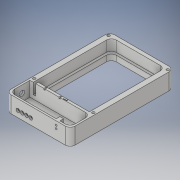
# Autodesk Inventor part: Bottom
Saved by Autodesk Inventor 2019 (Build 230136000, 136)
## iProperties
Created: 2020-07-16
Part Number: Bottom
Material: Generic
Document SubType Name: Modeling
Designer: Erle
Density: 1 g/cm^3
Appearance: Default
Author: Erle
Autodesk Inventor part; units mm, degrees
ref_plane "YZ Plane" through (0, 0, 0) normal (1, 0, 0) x (0, 1, 0)
ref_plane "XZ Plane" through (0, 0, 0) normal (0, 1, 0) x (-1, 0, 0)
ref_plane "XY Plane" through (0, 0, 0) normal (0, 0, 1) x (1, 0, 0)
sketch "Sketch1" plane through (0, 0, 0) normal (0, 1, 0) x (-1, 0, 0)
  line L0 (-52.5, 85) -> (52.5, 85)
  line L1 (52.5, 85) -> (52.5, -85)
  line L2 (52.5, -85) -> (-52.5, -85)
  line L3 (-52.5, -85) -> (-52.5, 85)
  line L4 (-52.5, 85) -> (52.5, -85) construction
  line L5 (52.5, 85) -> (-52.5, -85) construction
  line L6 (40, 45) -> (-40, 45)
  line L7 (-40, 45) -> (-40, -75)
  line L8 (-40, -75) -> (40, -75)
  line L9 (40, -75) -> (40, 45)
  point P0 (0, 0)
  point P1 (0, -75)
  point P2 (0, 0)
  point P3 (0, -85)
  dimension "d0" = 120
  dimension "d1" = 80
  dimension "d2" = 105
  dimension "d3" = 10
  dimension "d4" = 170
  constraints: 20 end point, 5 midpoint, 4 parallel, 2 horizontal, 2 perpendicular, 2 vertical alignment
  measures "d0" distance of L6.end L7.end
  measures "d1" distance of L7.end L8.end
  measures "d2" distance of L1.end L2.end
  measures "d3" distance between parallel lines of L2 L8
  measures "d4" distance of L0.end L1.end
extrude "Extrusion1" add sketch "Sketch1" along normal mid plane 27
sketch "Sketch2" plane through (0, 0, 0) normal (0, 1, 0) x (-1, 0, 0)
  line L0 (44, -79) -> (-44, -79)
  line L1 (-44, -79) -> (-44, 45)
  line L2 (-44, 45) -> (44, 45)
  line L3 (44, 45) -> (44, -79)
  line L4 (-40, -75) -> (40, -75) projected
  line L5 (40, -75) -> (40, 45) projected
  line L6 (-40, 45) -> (-40, -75) projected
  point P0 (0, 0)
  dimension "d7" = 4
  dimension "d8" = 4
  dimension "d9" = 4
  constraints: 8 end point, 2 parallel, 1 horizontal, 1 horizontal alignment, 1 perpendicular
  measures "d7" distance between parallel lines of L4 L0
  measures "d8" distance between parallel lines of L5 L3
  measures "d9" distance between parallel lines of L6 L1
extrude "Extrusion2" cut sketch "Sketch2" along normal blind 15 and the other way blind 4
sketch "Sketch3" plane through (0, 13.5, 0) normal (0, 1, 0) x (1, 0, 0)
  line L0 (-49.5, -49) -> (49.5, -49)
  line L1 (49.5, -49) -> (49.5, -82)
  line L2 (49.5, -82) -> (-49.5, -82)
  line L3 (-49.5, -82) -> (-49.5, -49)
  line L4 (-52.5, 85) -> (-52.5, -85) projected
  line L5 (-52.5, -85) -> (52.5, -85) projected
  line L6 (44, -45) -> (-44, -45) projected
  point P0 (0, 0)
  point P1 (0, -49)
  dimension "d14" = 3
  dimension "d15" = 3
  dimension "d16" = 4
  constraints: 8 end point, 2 parallel, 1 horizontal, 1 midpoint, 1 perpendicular, 1 vertical alignment
  measures "d14" distance between parallel lines of L4 L3
  measures "d15" distance between parallel lines of L5 L2
  measures "d16" distance between parallel lines of L6 L0
extrude "Extrusion3" cut sketch "Sketch3" against normal blind 24
sketch "Sketch4" plane through (0, 13.5, 0) normal (0, 1, 0) x (1, 0, 0)
  line L0 (44, -45) -> (-44, -45) projected
  line L1 (-49.5, -49) -> (49.5, -49) projected
  line L2 (-44, -45) -> (-40, -45)
  line L3 (-40, -45) -> (-40, -49)
  line L4 (-40, -49) -> (-44, -49)
  line L5 (-44, -49) -> (-44, -45)
  point P0 (0, 0)
  point P1 (-40, 75)
  constraints: 8 end point, 2 parallel, 1 horizontal, 1 perpendicular, 1 point on line, 1 vertical alignment
extrude "Extrusion4" cut sketch "Sketch4" against normal up to surface (17.5 mm away)
sketch "Sketch5" plane through (0, 13.5, 0) normal (0, 1, 0) x (1, 0, 0)
  line L0 (44, -45) -> (-40, -45) projected
  line L1 (-26.6, -48) -> (-24.7, -48)
  line L2 (-24.7, -48) -> (-24.7, -45)
  line L3 (-24.7, -45) -> (-26.6, -45)
  line L4 (-26.6, -45) -> (-26.6, -48)
  line L5 (-1.9, -48) -> (0, -48)
  line L6 (0, -48) -> (0, -45)
  line L7 (0, -45) -> (-1.9, -45)
  line L8 (-1.9, -45) -> (-1.9, -48)
  line L9 (-40, -45) -> (40, -45) projected
  point P0 (0, 0)
  dimension "d21" = 1.9
  dimension "d22" = 1.9
  dimension "d23" = 22.8
  dimension "d24" = 3
  constraints: 16 end point, 4 parallel, 3 point on line, 2 horizontal, 2 perpendicular, 1 midpoint, 1 vertical alignment
  measures "d21" distance of L1.start L1.end
  measures "d22" distance of L5.start L5.end
  measures "d23" distance between parallel lines of L8 L2
  measures "d24" distance of L3.end L1.start
extrude "Extrusion5" cut sketch "Sketch5" against normal blind 14
sketch "Sketch6" plane through (0, 13.5, 0) normal (0, 1, 0) x (1, 0, 0)
  line L0 (-40, -45) -> (40, -45) projected
  line L1 (9, -45) -> (9, -47.3)
  line L2 (9, -47.3) -> (3.7, -47.3)
  line L3 (3.7, -47.3) -> (3.7, -48)
  line L4 (3.7, -48) -> (9.7, -48)
  line L5 (9.7, -48) -> (9.7, -45)
  line L6 (0, -45) -> (0, -48) projected
  point P0 (0, 0)
  dimension "d27" = 0.7
  dimension "d28" = 0.7
  dimension "d29" = 3
  dimension "d30" = 6
  dimension "d31" = 9
  constraints: 10 end point, 4 perpendicular, 2 point on line, 1 vertical
  measures "d27" distance between parallel lines of L4 L2
  measures "d28" distance between parallel lines of L5 L1
  measures "d29" distance of L4.end L5.end
  measures "d30" distance of L3.end L4.end
  measures "d31" distance from line of L6 L1.start
extrude "Extrusion6" cut sketch "Sketch6" against normal blind 15
fillet "Fillet1" radius 8 12 edges at (-44, 4.75, -79) (44, 4.75, -79) (40, -8.75, -75) (-40, -8.75, -75) (52.5, 0, -85) (-52.5, 0, -85) (-52.5, 0, 85) (-49.5, 1.5, 82) (49.5, 1.5, 82) (52.5, 0, 85) (40, -8.75, 45) (-40, -8.75, 45)
sketch "Sketch7" plane through (0, -10.5, 0) normal (0, 1, 0) x (1, 0, 0)
  line L0 (-36, -74) -> (36, -74)
  line L1 (36, -74) -> (36, -72)
  line L2 (36, -72) -> (-36, -72)
  line L3 (-36, -72) -> (-36, -74)
  line L4 (41.5, -82) -> (-41.5, -82) projected
  point P0 (0, 0)
  point P1 (0, -72)
  dimension "d35" = 2
  dimension "d36" = 72
  dimension "d37" = 8
  constraints: 8 end point, 2 parallel, 1 horizontal, 1 midpoint, 1 perpendicular, 1 vertical alignment
  measures "d35" distance of L0.end L1.end
  measures "d36" distance of L1.end L2.end
  measures "d37" distance between parallel lines of L4 L0
extrude "Extrusion7" cut sketch "Sketch7" against normal blind 2
sketch "Sketch8" plane through (-52.5, -13.5, 77) normal (-1, 0, 0) x (0, 0, 1)
  line L0 (0, 0) -> (-154, 0) projected
  line L1 (-3, 3) -> (-3, 27) projected
  point P0 (-77, 13.5)
  point P1 (-15, 15)
  dimension "d40" = 15
  dimension "d41" = 12
  measures "d40" distance from line of L0 point (-15, 15)
  measures "d41" distance from line of L1 point (-15, 15)
hole "Hole1" at (-52.5, 1.5, 62) direction (1, 0, 0) diameter 8.4 depth 8 tip angle 118
fillet "Fillet2" radius 8 1 edges at (49.5, 1.5, 49)
sketch "Sketch9" plane through (0, 13.5, 0) normal (0, 1, 0) x (1, 0, 0)
  line L0 (-48.5, 79) -> (48.5, 79) construction
  line L1 (48.5, 79) -> (48.5, -43) construction
  line L2 (48.5, -43) -> (-48.5, -43) construction
  line L3 (-48.5, -43) -> (-48.5, 79) construction
  line L4 (44.5, 85) -> (-44.5, 85) projected
  line L5 (-52.5, 77) -> (-52.5, -77) projected
  line L6 (-40, -49) -> (41.5, -49) projected
  point P0 (0, 0)
  point P1 (0, 79)
  dimension "d50" = 6
  dimension "d51" = 4
  dimension "d52" = 6
  constraints: 8 end point, 4 coincident, 2 parallel, 1 horizontal, 1 midpoint, 1 perpendicular, 1 vertical alignment
  measures "d50" distance between parallel lines of L4 L0
  measures "d51" distance between parallel lines of L5 L3
  measures "d52" distance between parallel lines of L6 L2
hole "Hole2" at (-48.5, 13.5, -79) at (48.5, 13.5, -79) at (48.5, 13.5, 43) at (-48.5, 13.5, 43) direction (0, -1, 0) diameter 4.3 depth 8
sketch "Sketch10" plane through (-44.5, 13.5, 85) normal (0, 0, 1) x (1, 0, 0)
  circle A0 centre (25.3, -16.6) radius 3
  circle A1 centre (32.3, -16.6) radius 3
  circle A2 centre (18.3, -16.6) radius 3
  circle A3 centre (11.3, -16.6) radius 3
  line L0 (-8, 0) -> (-8, -27) projected
  line L1 (89, -27) -> (0, -27) projected
  point P0 (44.5, -13.5)
  dimension "d60" = 6
  dimension "d61" = 6
  dimension "d62" = 6
  dimension "d63" = 6
  dimension "d64" = 7
  dimension "d65" = 7
  dimension "d66" = 7
  dimension "d67" = 19.3
  dimension "d68" = 10.4
  constraints: 4 centre point, 3 horizontal alignment
  measures "d60" diameter of A0
  measures "d61" diameter of A1
  measures "d62" diameter of A2
  measures "d63" diameter of A3
  measures "d64" distance of A2.centre A3.centre
  measures "d65" distance of A1.centre A0.centre
  measures "d66" distance of A2.centre A0.centre
  measures "d67" distance from line of A3.centre L0
  measures "d68" distance from line of L1 A3.centre
extrude "Extrusion8" cut sketch "Sketch10" against normal blind 10
sketch "Sketch13" plane through (0, -10.5, 0) normal (0, 1, 0) x (1, 0, 0)
  line L0 (41.5, -82) -> (-41.5, -82) projected
  line L1 (26.65, -82) -> (32.65, -82)
  line L2 (32.65, -82) -> (32.65, -76)
  line L3 (32.65, -76) -> (26.65, -76)
  line L4 (26.65, -76) -> (26.65, -82)
  point P0 (0, 0)
  point P1 (52.5, -77)
  dimension "d78" = 6
  dimension "d79" = 6
  dimension "d82" = 19.85
  constraints: 8 end point, 2 parallel, 1 horizontal, 1 perpendicular, 1 point on line
  measures "d78" distance of L2.end L3.end
  measures "d79" distance of L1.end L2.end
  measures "d82" distance from line of point (52.5, -77) L2
extrude "Extrusion10" add sketch "Sketch13" along normal up to surface (24 mm away)
sketch "Sketch11" plane through (-44.5, 13.5, 85) normal (0, 0, 1) x (1, 0, 0)
  circle A0 centre (74.15, -11.19) radius 1.5
  circle A1 centre (74.15, -6.19) radius 1.5
  line L0 (89, -27) -> (0, -27) projected
  line L1 (97, -27) -> (97, 0) projected
  point P0 (44.5, -13.5)
  dimension "d71" = 3
  dimension "d72" = 3
  dimension "d73" = 5
  dimension "d76" = 20.81
  dimension "d77" = 22.85
  constraints: 2 centre point, 1 vertical alignment
  measures "d71" diameter of A0
  measures "d72" diameter of A1
  measures "d73" distance of A0.centre A1.centre
  measures "d76" distance from line of L0 A1.centre
  measures "d77" distance from line of A1.centre L1
extrude "Extrusion9" cut sketch "Sketch11" against normal blind 10
sketch "Sketch14" plane through (0, 13.5, 0) normal (0, 1, 0) x (1, 0, 0)
  line L0 (-24.7, -48) -> (-26.6, -48) projected
  line L1 (-40, -49) -> (41.5, -49) projected
  line L2 (-26.6, -48) -> (-24.7, -48)
  line L3 (-24.7, -48) -> (-24.7, -49)
  line L4 (-24.7, -49) -> (-26.6, -49)
  line L5 (-26.6, -49) -> (-26.6, -48)
  line L6 (0, -48) -> (-1.9, -48) projected
  line L7 (-1.9, -48) -> (0, -48)
  line L8 (0, -48) -> (0, -49)
  line L9 (0, -49) -> (-1.9, -49)
  line L10 (-1.9, -49) -> (-1.9, -48)
  point P0 (0, 0)
  constraints: 16 end point, 4 parallel, 2 horizontal, 2 perpendicular, 2 point on line, 1 coincident, 1 vertical alignment
extrude "Extrusion11" cut sketch "Sketch14" against normal blind 2
body "Solid1"
